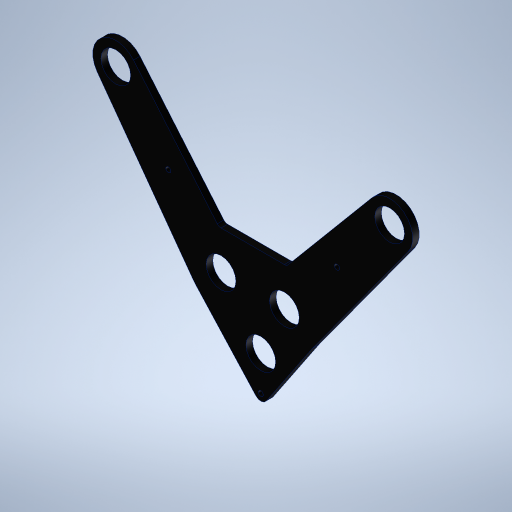
# Autodesk Inventor part: topplate_gearbox3_
Saved by Autodesk Inventor 2024 (Build 280153000, 153)
## iProperties
Created: 2024-12-21
Part Number: topplate_gearbox3_
Material: Aluminum 6061
Document SubType Name: Modeling
Designer: Danielle
Density: 2.7 g/cm^3
Appearance: Aluminum - Flat
Author: Danielle
Autodesk Inventor part; units mm, degrees
ref_plane "YZ Plane" through (0, 0, 0) normal (1, 0, 0) x (0, 1, 0)
ref_plane "XZ Plane" through (0, 0, 0) normal (0, 1, 0) x (-1, 0, 0)
ref_plane "XY Plane" through (0, 0, 0) normal (0, 0, 1) x (1, 0, 0)
sketch "Sketch1" plane through (0, 0, 0) normal (0, 0, 1) x (1, 0, 0)
  circle A0 centre (0, 0) radius 22.86 construction
  circle A1 centre (22.6979, 48.2696) radius 30.48 construction
  circle A2 centre (-38.2621, 48.2696) radius 30.48 construction
  circle A3 centre (0, 0) radius 25.4 construction
  circle A4 centre (22.6979, 48.2696) radius 33.02 construction
  circle A5 centre (-38.2621, 48.2696) radius 33.02 construction
  line L0 (-15.7782, 19.905) -> (-17.7504, 22.3931)
  circle A6 centre (-38.2621, 48.2696) radius 14.2875
  circle A7 centre (22.6979, 48.2696) radius 14.2875
  circle A8 centre (0, 0) radius 14.2875
  circle A9 centre (22.6979, 48.2696) radius 21.0058 construction
  circle A10 centre (22.6979, 48.2696) radius 19.1008 construction
  circle A11 centre (-38.2621, 48.2696) radius 19.1008 construction
  circle A12 centre (-38.2621, 48.2696) radius 21.0058 construction
  line L1 (22.6979, 48.2696) -> (123.9969, 169.1436) construction
  circle A13 centre (-139.561, 169.1436) radius 14.2875
  circle A14 centre (123.9969, 169.1436) radius 14.2875
  line L2 (-139.561, 169.1436) -> (-38.2621, 48.2696) construction
  circle A15 centre (-139.561, 169.1436) radius 22.225 construction
  circle A16 centre (123.9969, 169.1436) radius 22.225 construction
  line L3 (-122.5269, 183.4191) -> (-41.9122, 87.2264)
  arc A17 (-41.9122, 87.2264) -> (-38.2621, 85.523) centre (-38.2621, 90.2855) ccw
  line L4 (-38.2621, 85.523) -> (22.6979, 85.523)
  arc A18 (22.6979, 85.523) -> (26.3481, 87.2264) centre (22.6979, 90.2855) ccw
  line L5 (26.3481, 87.2264) -> (106.9628, 183.4191)
  line L6 (-38.2621, 81.2896) -> (-38.2621, 85.523) construction
  line L7 (22.6979, 81.2896) -> (22.6979, 85.523) construction
  arc A19 (-122.5269, 183.4191) -> (-157.5323, 156.0676) centre (-139.561, 169.1436) ccw
  circle A20 centre (-88.9115, 108.7066) radius 2.4892
  circle A21 centre (73.3474, 108.7066) radius 2.4892
  circle A22 centre (-88.9115, 108.7066) radius 6.35 construction
  circle A23 centre (73.3474, 108.7066) radius 6.35 construction
  line L8 (-157.5323, 156.0676) -> (-64.9623, 28.8424)
  circle A24 centre (0, -33.3375) radius 6.35 construction
  circle A25 centre (0, -33.3375) radius 2.4892
  line L9 (0, -26.9875) -> (0, -25.4) construction
  line L10 (-62.6725, 26.0334) -> (-4.6943, -37.6137)
  arc A26 (-64.9623, 28.8424) -> (-62.6725, 26.0334) centre (-38.2621, 48.2696) ccw
  line L11 (5.2709, -36.8788) -> (50.1064, 29.8551)
  arc A27 (-4.6943, -37.6137) -> (5.2709, -36.8788) centre (0, -33.3375) ccw
  arc A28 (141.9682, 156.0676) -> (106.9628, 183.4191) centre (123.9969, 169.1436) ccw
  line L12 (141.9682, 156.0676) -> (49.3982, 28.8424)
  line L13 (50.1064, 29.8551) -> (49.3982, 28.8424)
  circle A29 centre (-139.561, 169.1436) radius 50.8 construction
  circle A30 centre (123.9969, 169.1436) radius 50.8 construction
  point P0 (-38.2621, 83.4063)
  point P1 (49.7618, 29.3421)
  dimension "d0" = 45.72
  dimension "d1" = 60.96
  dimension "d2" = 2.54
  dimension "d3" = 2.54
  dimension "d4" = 3.175
  dimension "d5" = 28.575
  dimension "d6" = 42.0116
  dimension "d7" = 38.2016
  dimension "d14" = 44.45
  dimension "d15" = 44.45
  dimension "d16" = 4.7625
  dimension "d17" = 4.2333
  dimension "d18" = 4.9784
  dimension "d19" = 4.9784
  dimension "d20" = 12.7
  dimension "d21" = 12.7
  dimension "d23" = 1.5875
  dimension "d24" = 157.7086
  dimension "d25" = 101.6
  dimension "d26" = 101.6
  constraints: 31 centre point, 28 end point, 28 point on circle, 20 tangent, 16 coincident, 14 equal radius, 7 point on line, 3 midpoint, 2 concentric, 2 equal length, 2 horizontal alignment, 2 parallel, 2 perpendicular, 1 horizontal, 1 vertical, 1 vertical alignment
  measures "d0" diameter of A0
  measures "d1" diameter of A1
  measures "d2" radial gap between concentric circles of A0 A3
  measures "d3" radial gap between concentric circles of A1 A4
  measures "d4" distance of L0.start L0.end
  measures "d5" diameter of A6
  measures "d6" diameter of A9
  measures "d7" diameter of A10
  measures "d14" diameter of A15
  measures "d15" diameter of A16
  measures "d16" radius of A17
  measures "d17" distance of L6.start L6.end
  measures "d18" diameter of A20
  measures "d19" diameter of A21
  measures "d20" diameter of A22
  measures "d21" diameter of A23
  measures "d23" distance of L9.start L9.end
  measures "d24" distance of L2.start L2.end
  measures "d25" diameter of A29
  measures "d26" diameter of A30
extrude "Extrusion1" add sketch "Sketch1" along normal blind 6.35 contours L12 L13 L11 | L3 A17 L4 A18 L5 A28 L12 L11 A27 L10 A26 L8 A19
body "Solid1"
